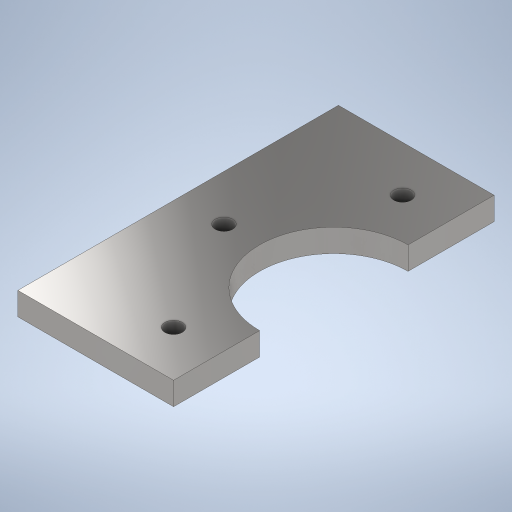
# Autodesk Inventor part: sguard
Saved by Autodesk Inventor 2023 (Build 270158000, 158)
## iProperties
Created: 2023-03-12
Part Number: sguard
Material: Steel, High Strength, Low Alloy
Document SubType Name: Modeling
Designer: William Allport
Density: 7.85 g/cm^3
Appearance: Steel - Polished
Author: William Allport
Autodesk Inventor part; units mm, degrees
ref_plane "YZ Plane" through (0, 0, 0) normal (1, 0, 0) x (0, 1, 0)
ref_plane "XZ Plane" through (0, 0, 0) normal (0, 1, 0) x (-1, 0, 0)
ref_plane "XY Plane" through (0, 0, 0) normal (0, 0, 1) x (1, 0, 0)
sketch "Sketch1" plane through (0, 0, 0) normal (0, 1, 0) x (-1, 0, 0)
  line L0 (0, 0) -> (-43.18, 0)
  line L1 (-43.18, 0) -> (-43.18, 88.9)
  line L2 (-43.18, 88.9) -> (0, 88.9)
  line L3 (0, 88.9) -> (0, 0)
  dimension "d0" = 43.18
  dimension "d1" = 88.9
  constraints: 8 end point, 2 parallel, 1 horizontal, 1 perpendicular
  measures "d0" distance of L1.end L2.end
  measures "d1" distance of L0.end L1.end
extrude "Extrusion1" add sketch "Sketch1" along normal blind 6.35
sketch "Sketch2" plane through (0, 6.35, 0) normal (0, 1, 0) x (1, 0, 0)
  line L0 (0, 0) -> (0, -88.9) projected
  line L1 (43.18, 0) -> (0, 0) projected
  point P0 (43.18, -44.45)
  dimension "d4" = 43.18
  dimension "d5" = 44.45
  measures "d4" distance from line of L0 point (43.18, -44.45)
  measures "d5" distance from line of L1 point (43.18, -44.45)
hole "Hole1" at (43.18, 6.35, 44.45) direction (0, -1, 0) diameter 41.148 end through all
sketch "Sketch3" plane through (0, 6.35, 0) normal (0, 1, 0) x (1, 0, 0)
  line L0 (43.18, -23.876) -> (43.18, 0) projected
  line L1 (43.18, 0) -> (0, 0) projected
  point P0 (12.7, -44.45)
  dimension "d13" = 30.48
  dimension "d14" = 44.45
  measures "d13" distance from line of L0 point (12.7, -44.45)
  measures "d14" distance from line of L1 point (12.7, -44.45)
hole "Hole2" at (12.7, 6.35, 44.45) direction (0, -1, 0) diameter 4.826 end through all
sketch "Sketch4" plane through (0, 6.35, 0) normal (0, 1, 0) x (1, 0, 0)
  line L0 (43.18, -23.876) -> (43.18, 0) projected
  line L1 (43.18, 0) -> (0, 0) projected
  point P0 (30.48, -12.7)
  dimension "d22" = 12.7
  dimension "d23" = 12.7
  measures "d22" distance from line of L0 point (30.48, -12.7)
  measures "d23" distance from line of L1 point (30.48, -12.7)
hole "Hole3" at (30.48, 6.35, 12.7) direction (0, -1, 0) diameter 4.826 end through all
sketch "Sketch6" plane through (0, 6.35, 0) normal (0, 1, 0) x (1, 0, 0)
  line L0 (43.18, -88.9) -> (43.18, -65.024) construction
  line L1 (0, -88.9) -> (43.18, -88.9) construction
  point P0 (0, 0)
  point P1 (30.48, -76.2)
  dimension "d50" = 12.7
  dimension "d51" = 12.7
  measures "d50" distance from line of L0 point (30.48, -76.2)
  measures "d51" distance from line of L1 point (30.48, -76.2)
hole "Hole5" at (30.48, 6.35, 76.2) direction (0, -1, 0) diameter 4.826 end through all
body "Solid1"
